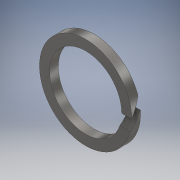
# Autodesk Inventor part: PistonRing
Saved by Autodesk Inventor 2017 (Build 210142000, 142)
## iProperties
Created: 2018-11-05
Part Number: PistonRing
Material: Stainless Steel
Document SubType Name: Modeling
Designer: 623516
Density: 8 g/cm^3
Appearance: Semi-Polished
Author: 623516
Autodesk Inventor part; units mm, degrees
ref_plane "XZ Plane" through (0, 0, 0) normal (0, 1, 0) x (-1, 0, 0)
ref_plane "XY Plane" through (0, 0, 0) normal (0, 0, 1) x (1, 0, 0)
sketch "Sketch1" plane through (0, 0, 0) normal (0, 1, 0) x (-1, 0, 0)
  circle A0 centre (0, 0) radius 16
  circle A1 centre (0, 0) radius 12.5
  dimension "d0" = 32
  dimension "d1" = 25
  constraints: 2 centre point, 2 coincident
  measures "d0" diameter of A0
  measures "d1" diameter of A1
extrude "Extrusion1" add sketch "Sketch1" along normal blind 3
ref_plane "Work Plane1" through (16.25, 0, 0) normal (1, 0, 0) x (0, 1, 0)
sketch "Sketch2" plane through (16.25, 0, 0) normal (1, 0, 0) x (0, 1, 0)
  line L0 (0, 0) -> (3, 5.1962)
  line L1 (3, -16) -> (3, 16) projected
  line L2 (0, -12.5) -> (0, 12.5) projected
  line L3 (0, 0) -> (0, -4)
  line L4 (0, 16) -> (0, -16) projected
  line L5 (0, -4) -> (3, 1.1962)
  line L6 (3, 5.1962) -> (3, 1.1962)
  dimension "d10" = 2
  dimension "d11" = 30
  constraints: 8 end point, 3 point on line, 1 collinear
  measures "d10" distance between parallel lines of L5 L0
  measures "d11" angle of L0 L2
extrude "Extrusion2" cut sketch "Sketch2" against normal blind 9
body "Solid1"
